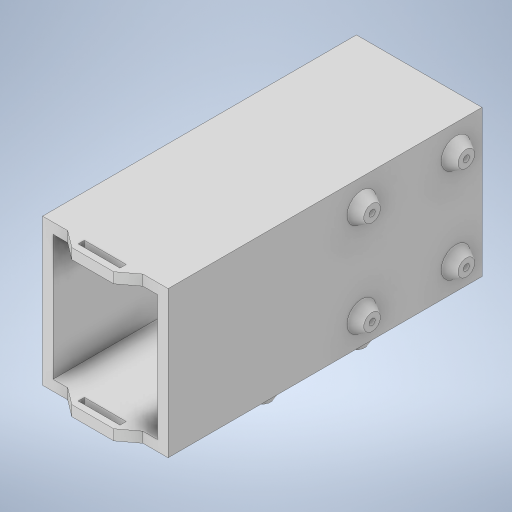
# Autodesk Inventor part: Battery Mount - EthanMockup
Saved by Autodesk Inventor 2023 (Build 270158000, 158)
## iProperties
Created: 2023-01-11
Part Number: Battery Mount - EthanMockup
Material: Generic
Document SubType Name: Modeling
Designer: Administrator
Density: 1 g/cm^3
Appearance: Default
Author: Administrator
Autodesk Inventor part; units mm, degrees
ref_plane "YZ Plane" through (0, 0, 0) normal (1, 0, 0) x (0, 1, 0)
ref_plane "XZ Plane" through (0, 0, 0) normal (0, 1, 0) x (-1, 0, 0)
ref_plane "XY Plane" through (0, 0, 0) normal (0, 0, 1) x (1, 0, 0)
sketch "Sketch1" plane through (0, 0, 0) normal (0, 0, 1) x (1, 0, 0)
  line L0 (0, 0) -> (50, 0)
  line L1 (50, 0) -> (50, 60)
  line L2 (50, 60) -> (0, 60)
  line L3 (0, 60) -> (0, 0)
  line L4 (-5, -5) -> (55, -5)
  line L5 (55, -5) -> (55, 65)
  line L6 (55, 65) -> (-5, 65)
  line L7 (-5, 65) -> (-5, -5)
  dimension "d0" = 50
  dimension "d1" = 60
  dimension "d2" = 5
  dimension "d3" = 5
  dimension "d4" = 5
  dimension "d5" = 5
  constraints: 16 end point, 4 parallel, 2 horizontal, 2 perpendicular
  measures "d0" distance of L2.end L1.end
  measures "d1" distance of L1.end L0.end
  measures "d2" distance between parallel lines of L3 L7
  measures "d3" distance between parallel lines of L5 L1
  measures "d4" distance between parallel lines of L4 L0
  measures "d5" distance between parallel lines of L6 L2
extrude "Extrusion1" add sketch "Sketch1" along normal blind 150 contours L3 L2 L1 L0 | L7 L6 L5 L4
sketch "Sketch2" plane through (-5, -5, 0) normal (-1, 0, 0) x (0, 0, 1)
  line L0 (150, 0) -> (150, 70) construction
  line L1 (0, 70) -> (150, 70) construction
  line L2 (150, 0) -> (80, 0) construction
  line L3 (80, 0) -> (80, 70) construction
  line L4 (80, 70) -> (150, 70) construction
  line L5 (150, 70) -> (150, 0) construction
  line L6 (80, 70) -> (150, 0) construction
  line L7 (150, 70) -> (80, 0) construction
  line L8 (92.5, 12.5) -> (137.5, 12.5) construction
  line L9 (137.5, 12.5) -> (137.5, 57.5) construction
  line L10 (137.5, 57.5) -> (92.5, 57.5) construction
  line L11 (92.5, 57.5) -> (92.5, 12.5) construction
  line L12 (92.5, 12.5) -> (137.5, 57.5) construction
  line L13 (137.5, 12.5) -> (92.5, 57.5) construction
  circle A0 centre (92.5, 57.5) radius 4
  circle A1 centre (137.5, 57.5) radius 4
  circle A2 centre (137.5, 12.5) radius 4
  circle A3 centre (92.5, 12.5) radius 4
  circle A4 centre (92.5, 57.5) radius 1.5
  circle A5 centre (137.5, 57.5) radius 1.5
  circle A6 centre (137.5, 12.5) radius 1.5
  circle A7 centre (92.5, 12.5) radius 1.5
  point P0 (0, 5)
  point P1 (115, 35)
  dimension "d10" = 70
  dimension "d11" = 45
  dimension "d12" = 45
  dimension "d13" = 8
  dimension "d14" = 8
  dimension "d15" = 8
  dimension "d16" = 8
  dimension "d19" = 3
  dimension "d20" = 3
  dimension "d21" = 3
  dimension "d22" = 3
  constraints: 24 end point, 8 centre point, 8 coincident, 4 parallel, 3 midpoint, 2 horizontal, 2 perpendicular, 1 point on line
  measures "d10" distance of L3.end L4.end
  measures "d11" distance of L10.end L9.end
  measures "d12" distance of L9.end L8.end
  measures "d13" diameter of A0
  measures "d14" diameter of A1
  measures "d15" diameter of A2
  measures "d16" diameter of A3
  measures "d19" diameter of A4
  measures "d20" diameter of A5
  measures "d21" diameter of A6
  measures "d22" diameter of A7
extrude "Extrusion3" add sketch "Sketch2" along normal blind 5
chamfer "Chamfer1" distance 3 distance2 5 4 edges at (-5, 7.5, 88.5) (-5, 52.5, 88.5) (-5, 52.5, 133.5) (-5, 7.5, 133.5) measured on face at (-5, 7.5, 88) measured on face at (-5, 7.5, 133) measured on face at (-5, 52.5, 88) measured on face at (-5, 52.5, 133)
sketch "Sketch3" plane through (-5, -5, 0) normal (0, -1, 0) x (1, 0, 0)
  line L0 (0, 0) -> (60, 0) construction
  line L1 (60, 150) -> (0, 150) construction
  line L2 (0, 0) -> (60, 150) construction
  line L3 (52.5, 52.5) -> (7.5, 52.5) construction
  line L4 (7.5, 52.5) -> (7.5, 97.5) construction
  line L5 (7.5, 97.5) -> (52.5, 97.5) construction
  line L6 (52.5, 97.5) -> (52.5, 52.5) construction
  line L7 (52.5, 52.5) -> (7.5, 97.5) construction
  line L8 (7.5, 52.5) -> (52.5, 97.5) construction
  circle A0 centre (7.5, 52.5) radius 4
  circle A1 centre (7.5, 97.5) radius 4
  circle A2 centre (52.5, 97.5) radius 4
  circle A3 centre (52.5, 52.5) radius 4
  circle A4 centre (52.5, 52.5) radius 1.5
  circle A5 centre (7.5, 52.5) radius 1.5
  circle A6 centre (7.5, 97.5) radius 1.5
  circle A7 centre (52.5, 97.5) radius 1.5
  point P0 (5, 0)
  point P1 (30, 75)
  dimension "d26" = 45
  dimension "d27" = 45
  dimension "d28" = 8
  dimension "d29" = 8
  dimension "d30" = 8
  dimension "d31" = 8
  dimension "d32" = 3
  dimension "d33" = 3
  dimension "d34" = 3
  dimension "d35" = 3
  constraints: 14 end point, 8 centre point, 8 coincident, 3 midpoint, 2 parallel, 1 horizontal, 1 perpendicular
  measures "d26" distance of L4.end L5.end
  measures "d27" distance of L3.end L4.end
  measures "d28" diameter of A0
  measures "d29" diameter of A1
  measures "d30" diameter of A2
  measures "d31" diameter of A3
  measures "d32" diameter of A4
  measures "d33" diameter of A5
  measures "d34" diameter of A6
  measures "d35" diameter of A7
extrude "Extrusion4" add sketch "Sketch3" along normal blind 5
chamfer "Chamfer2" distance 3 distance2 5 4 edges at (43.5, -5, 52.5) (-1.5, -5, 52.5) (-1.5, -5, 97.5) (43.5, -5, 97.5) measured on face at (43, -5, 97.5) measured on face at (43, -5, 52.5) measured on face at (-2, -5, 52.5) measured on face at (-2, -5, 97.5)
sketch "Sketch4" plane through (55, -5, 0) normal (1, 0, 0) x (0, 0, -1)
  line L0 (0, 70) -> (-150, 70) construction
  line L1 (0, 0) -> (0, 70) construction
  line L2 (-150, 70) -> (0, 0) construction
  line L3 (-140, 10) -> (-10, 10) construction
  line L4 (-10, 10) -> (-10, 60) construction
  line L5 (-10, 60) -> (-140, 60) construction
  line L6 (-140, 60) -> (-140, 10) construction
  line L7 (-140, 10) -> (-10, 60) construction
  line L8 (-10, 10) -> (-140, 60) construction
  circle A0 centre (-140, 60) radius 4
  circle A1 centre (-140, 10) radius 4
  circle A2 centre (-10, 10) radius 4
  circle A3 centre (-10, 60) radius 4
  circle A4 centre (-140, 60) radius 1.5
  circle A5 centre (-140, 10) radius 1.5
  circle A6 centre (-10, 10) radius 1.5
  circle A7 centre (-10, 60) radius 1.5
  point P0 (0, 5)
  point P1 (-75, 35)
  dimension "d41" = 130
  dimension "d42" = 50
  dimension "d43" = 8
  dimension "d44" = 8
  dimension "d45" = 8
  dimension "d46" = 8
  dimension "d47" = 3
  dimension "d48" = 3
  dimension "d49" = 3
  dimension "d50" = 3
  constraints: 14 end point, 8 centre point, 8 coincident, 3 midpoint, 2 parallel, 1 horizontal, 1 perpendicular
  measures "d41" distance of L5.end L4.end
  measures "d42" distance of L4.end L3.end
  measures "d43" diameter of A0
  measures "d44" diameter of A1
  measures "d45" diameter of A2
  measures "d46" diameter of A3
  measures "d47" diameter of A4
  measures "d48" diameter of A5
  measures "d49" diameter of A6
  measures "d50" diameter of A7
extrude "Extrusion5" add sketch "Sketch4" along normal blind 5
chamfer "Chamfer3" distance 3 distance2 5 4 edges at (55, 55, 144) (55, 5, 144) (55, 5, 14) (55, 55, 14) measured on face at (55, 55, 144.5) measured on face at (55, 5, 14.5) measured on face at (55, 5, 144.5) measured on face at (55, 55, 14.5)
sketch "Sketch5" plane through (-5, -5, 0) normal (0, -1, 0) x (1, 0, 0)
  line L0 (5, 0) -> (55, 0) projected
  line L1 (40, 0) -> (20, 0)
  line L2 (20, 0) -> (20, -3)
  line L3 (20, -3) -> (40, -3)
  line L4 (40, -3) -> (40, 0)
  line L5 (0, 0) -> (0, 150) projected
  line L6 (60, 0) -> (60, 150) projected
  line L7 (40, 0) -> (48, 0)
  line L8 (20, 0) -> (12, 0)
  line L9 (40, -3) -> (40, -6) construction
  line L10 (48, 0) -> (40, -6)
  line L11 (40, -6) -> (20, -6)
  line L12 (20, -6) -> (12, 0)
  point P0 (20, 0)
  dimension "d56" = 20
  dimension "d57" = 3
  dimension "d58" = 60
  dimension "d59" = 20
  dimension "d60" = 8
  dimension "d61" = 8
  dimension "d62" = 3
  constraints: 20 end point, 3 point on line, 2 horizontal, 2 parallel, 1 perpendicular, 1 vertical
  measures "d56" distance of L3.end L2.end
  measures "d57" distance of L2.end L1.end
  measures "d58" distance between parallel lines of L5 L6
  measures "d59" distance of L6.start L1.start
  measures "d60" distance of L1.start L7.end
  measures "d61" distance of L1.end L8.end
  measures "d62" distance of L3.end L9.end
extrude "Extrusion6" add sketch "Sketch5" against normal blind 70 contours L0 L2 L3 L4 L10 L11 L12
extrude "Extrusion7" cut sketch "Sketch1" along normal blind 145 and the other way blind 6 contours L3 L2 L1 L0
equation "\"d59\" = -0.5 * d56 + 0.5 * d58"
body "Solid1"
